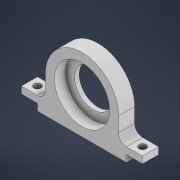
# Autodesk Inventor part: Halterung_Differential_2
Saved by Autodesk Inventor 2021 (Build 250183000, 183)
## iProperties
Created: 2021-01-24
Part Number: Halterung_Differential_2
Material: Generisch
Document SubType Name: Modeling
Designer: Ctroi
Density: 1 g/cm^3
Appearance: Vorgabe
Author: Ctroi
Autodesk Inventor part; units mm, degrees
ref_plane "YZ Plane" through (0, 0, 0) normal (1, 0, 0) x (0, 1, 0)
ref_plane "XZ Plane" through (0, 0, 0) normal (0, 1, 0) x (-1, 0, 0)
ref_plane "XY Plane" through (0, 0, 0) normal (0, 0, 1) x (1, 0, 0)
sketch "Skizze1" plane through (0, 0, 0) normal (0, 0, 1) x (1, 0, 0)
  line L0 (0, 22.4) -> (0, -22.4) projected
  line L1 (-22.4, 0) -> (22.4, 0) projected
  line L2 (-16, 16) -> (16, 16)
  line L3 (16, 16) -> (16, -16)
  line L4 (16, -16) -> (-16, -16)
  line L5 (-16, -16) -> (-16, 16)
  circle A0 centre (0, 0) radius 12.1
  dimension "d0" = 32
  dimension "d1" = 32
  dimension "d2" = 24.2
  constraints: 8 end point, 2 parallel, 1 centre point, 1 coincident, 1 horizontal, 1 perpendicular, 2 other
  measures "d0" distance of L3.end L4.end
  measures "d1" distance of L2.end L3.end
  measures "d2" diameter of A0
extrude "Extrusion1" add sketch "Skizze1" along normal blind 7 contours L2 L3 L1 A0 L0 | L0 A0 L1 L5 L2 | L1 L3 L4 L0 A0 | A0 L0 L4 L5 L1
sketch "Skizze2" plane through (16, -16, 0) normal (1, 0, 0) x (0, 0, -1)
  line L0 (-7, 32) -> (-7, 0) projected
  line L1 (0, 32) -> (0, 0) projected
  line L2 (-7, 0) -> (0, 0)
  line L3 (0, 0) -> (0, 6)
  line L4 (0, 6) -> (-7, 6)
  line L5 (-7, 6) -> (-7, 0)
  line L6 (0, 3) -> (-7, 3)
  point P0 (0, 16)
  point P1 (-7, 6)
  point P2 (0, 3)
  dimension "d5" = 6
  constraints: 10 end point, 2 midpoint, 2 parallel, 1 horizontal, 1 perpendicular, 1 point on line
  measures "d5" distance of L3.end L2.end
sketch "Skizze3" plane through (-16, -16, 0) normal (-1, 0, 0) x (0, 0, 1)
  line L0 (7, 32) -> (7, 0) projected
  line L1 (0, 32) -> (0, 0) projected
  line L2 (7, 0) -> (0, 0)
  line L3 (0, 0) -> (0, 6)
  line L4 (0, 6) -> (7, 6)
  line L5 (7, 6) -> (7, 0)
  line L6 (0, 3) -> (7, 3)
  point P0 (0, 16)
  point P1 (7, 6)
  point P2 (0, 3)
  point P3 (7, 3)
  dimension "d6" = 6
  constraints: 10 end point, 2 midpoint, 2 parallel, 1 horizontal, 1 perpendicular, 1 point on line
  measures "d6" distance of L2.end L3.end
sketch "Skizze4" plane through (0, 0, 0) normal (0, 0, -1) x (-1, 0, 0)
  circle A0 centre (0, 0) radius 12.1
  circle A1 centre (0, 0) radius 12.1 projected
  circle A2 centre (0, 0) radius 8.25
  dimension "d11" = 24.2
  dimension "d12" = 16.5
  constraints: 2 centre point, 2 coincident
  measures "d11" diameter of A0
  measures "d12" diameter of A2
extrude "Extrusion4" add sketch "Skizze4" against normal blind 2
fillet "Rundung1" radius 16 2 edges at (16, 16, 3.5) (-16, 16, 3.5)
extrude "Extrusion6" add sketch "Skizze3" along normal blind 10.5 contours L0 L6 L1 L4
extrude "Extrusion7" add sketch "Skizze2" along normal blind 10.5 contours L4 L1 L6 L0
sketch "Skizze6" plane through (16, -10, 7) normal (0, 1, 0) x (1, 0, 0)
  circle A0 centre (7, 3.5) radius 1.6
  line L0 (0, 7) -> (10.5, 7) projected
  line L1 (10.5, 7) -> (10.5, 0) projected
  circle A1 centre (-39, 3.5) radius 1.6
  line L2 (-42.5, 0) -> (-42.5, 7) projected
  line L3 (-32, 7) -> (-42.5, 7) projected
  point P0 (-16, 7)
  dimension "d29" = 3.2
  dimension "d30" = 3.5
  dimension "d31" = 3.5
  dimension "d32" = 3.2
  dimension "d33" = 3.5
  dimension "d34" = 3.5
  constraints: 2 centre point
  measures "d29" diameter of A0
  measures "d30" distance from line of L0 A0.centre
  measures "d31" distance from line of L1 A0.centre
  measures "d32" diameter of A1
  measures "d33" distance from line of L2 A1.centre
  measures "d34" distance from line of L3 A1.centre
extrude "Extrusion8" cut sketch "Skizze6" against normal up to surface (3 mm away)
sketch "Skizze7" plane through (16, -16, 7) normal (1, 0, 0) x (0, 0, -1)
  line L0 (7, 0) -> (0, 0) projected
  line L1 (0, 3) -> (0, 0) projected
  line L2 (7, 0) -> (0, 0)
  line L3 (0, 0) -> (0, 3)
  line L4 (0, 3) -> (7, 3)
  line L5 (7, 3) -> (7, 0)
  point P0 (7, 16)
  constraints: 8 end point, 2 parallel, 1 horizontal, 1 perpendicular
extrude "Extrusion9" add sketch "Skizze7" along normal blind 3.5
sketch "Skizze8" plane through (-16, -16, 0) normal (-1, 0, 0) x (0, 0, 1)
  line L0 (0, 0) -> (7, 0) projected
  line L1 (0, 0) -> (0, 3) projected
  line L2 (7, 0) -> (0, 0)
  line L3 (0, 0) -> (0, 3)
  line L4 (0, 3) -> (7, 3)
  line L5 (7, 3) -> (7, 0)
  point P0 (0, 16)
  constraints: 8 end point, 2 parallel, 1 horizontal, 1 perpendicular
extrude "Extrusion10" add sketch "Skizze8" along normal blind 3.5
fillet "Rundung3" radius 3.5 2 edges at (16, -10, 3.5) (-16, -10, 3.5)
